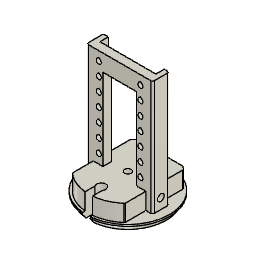
HANDLE_CONNECTOR v8 (Autodesk Fusion 360 design; units mm, degrees)
Autodesk Fusion 360 part; units mm, degrees
note: some values were not read from the file. Set by a fixed rule: which sketch regions a step uses.
sketch "Schizzo1" plane through (0, 0, 0) normal (0, 0, 1) x (1, 0, 0)
  circle A0 centre (0, 0) radius 25
  line L0 (0, 0) -> (0, 25) construction
  line L1 (0, 0) -> (0, -25) construction
  line L2 (-15.8, 19.3742) -> (-15.8, 17.5305) construction
  line L3 (-15.8, 17.5305) -> (-15.8, -17.5305)
  line L4 (-15.8, -17.5305) -> (-15.8, -19.3742) construction
  line L5 (15.8, 19.3742) -> (15.8, 17.5305) construction
  line L6 (15.8, 17.5305) -> (15.8, -17.5305)
  line L7 (15.8, -17.5305) -> (15.8, -19.3742) construction
  arc A1 (15.8, 17.5305) -> (-15.8, 17.5305) centre (0, 0) ccw
  arc A2 (-15.8, -17.5305) -> (15.8, -17.5305) centre (0, 0) ccw
  line L8 (-15.8, 0) -> (-19.8, 0) construction
  line L9 (15.8, 0) -> (19.8, 0) construction
  line L10 (-19.8, 0) -> (-19.8, 5)
  line L11 (-19.8, 5) -> (-15.8, 5)
  line L12 (-19.8, 0) -> (-19.8, -5)
  line L13 (-19.8, -5) -> (-15.8, -5)
  line L14 (19.8, 0) -> (19.8, 5)
  line L15 (19.8, 5) -> (15.8, 5)
  line L16 (19.8, 0) -> (19.8, -5)
  line L17 (19.8, -5) -> (15.8, -5)
  circle A3 centre (0, 0) radius 2
  circle A4 centre (0, -16) radius 2.75
  circle A5 centre (0, 10) radius 2
  line L18 (13.723, 19.2) -> (-13.723, 19.2)
  line L19 (2.25, -17.5811) -> (2.25, -24.8985)
  line L20 (-2.25, -17.5811) -> (-2.25, -24.8985)
  dimension "d1" = 50
  dimension "d3" = 31.6
  dimension "d4" = 1.4
  dimension "d5" = 10
  dimension "d6" = 4
  dimension "d21" = 4
  dimension "d22" = 5.5
  dimension "d23" = 16
  dimension "d39" = 4
  dimension "d40" = 10
  dimension "d45" = 5.8
  dimension "d48" = 4.5
  constraint coincident A0.centre L0.start
  constraint coincident A0 L0.end
  constraint vertical L0
  constraint coincident A0 L1.end
  constraint parallel L0 L1
  constraint coincident A0 L2.start
  constraint vertical L2
  constraint parallel L2 L3
  constraint coincident A0 L4.end
  constraint parallel L3 L4
  constraint coincident A0 L5.start
  constraint parallel L0 L5
  constraint parallel L5 L6
  constraint coincident A0 L7.end
  constraint parallel L6 L7
  constraint equal L5 L7
  constraint equal L2 L4
  constraint equal L2 L5
  constraint equal L3 L6
  constraint midpoint L3 L8.start
  constraint perpendicular L3 L8
  constraint midpoint L6 L9.start
  constraint perpendicular L6 L9
  constraint perpendicular L8 L10
  constraint coincident L3 L11.end
  constraint perpendicular L3 L11
  constraint perpendicular L8 L12
  constraint coincident L3 L13.end
  constraint perpendicular L3 L13
  constraint perpendicular L9 L14
  constraint coincident L6 L15.end
  constraint perpendicular L6 L15
  constraint perpendicular L9 L16
  constraint coincident L6 L17.end
  constraint perpendicular L6 L17
  constraint equal L10 L12
  constraint equal L14 L16
  constraint equal L12 L16
  constraint equal L8 L9
  constraint concentric A1 A3
  constraint coincident L1 A4.centre
  constraint coincident L0 A5.centre
  constraint coincident A1 L18.start
  constraint coincident A1 L18.end
  constraint perpendicular L6 L18
  constraint coincident A4 L19.start
  constraint coincident A0 L19.end
  constraint vertical L19
  constraint coincident A4 L20.start
  constraint coincident A0 L20.end
  constraint parallel L19 L20
  constraint equal L19 L20
  measures "d1" diameter of A0
  measures "d3" distance of L3 L6
  measures "d4" distance of A0 A1
  measures "d5" distance of L11 L13
  measures "d6" distance of L8.start L8.end
  measures "d21" diameter of A3
  measures "d22" diameter of A4
  measures "d23" distance of A0.centre A4.centre
  measures "d39" diameter of A5
  measures "d40" distance of A0.centre A5.centre
  measures "d45" distance of L0.end L18
  measures "d48" distance of L19 L20
extrude "Estrusione1" add sketch "Schizzo1" along normal blind 10 contours L3 L6 A1 A2 A4 L18 L19 L20 | L3 L10 L11 L12 L13 | L6 L14 L15 L16 L17
extrude "Estrusione2" add sketch "Schizzo1" against normal blind 4 contours A0 L3 L6 A1 A2 L10 L11 L12 L13 L14 L15 L16 L17 L19 L20 | L3 L6 A1 A2 A4 L18 L19 L20 | L3 L10 L11 L12 L13 | L6 L14 L15 L16 L17 | A1 L18
sketch "Schizzo2" plane through (-19.8, 0, 0) normal (-1, 0, 0) x (0, -1, 0)
  line L0 (-5, 0) -> (5, 0)
  line L1 (5, 0) -> (5, 10)
  line L2 (5, 10) -> (-5, 10)
  line L3 (-5, 10) -> (-5, 0)
  line L4 (0, 0) -> (0, 6.2) construction
  circle A0 centre (0, 6.2) radius 2
  dimension "d11" = 6.2
  dimension "d12" = 4
  constraint coincident L4.start origin
  constraint perpendicular L0 L4
  constraint coincident L4.end A0.centre
  measures "d11" distance of L4.start L4.end
  measures "d12" diameter of A0
extrude "Estrusione3" cut sketch "Schizzo2" against normal blind 15 contours A0
sketch "Schizzo3" plane through (19.8, 0, 0) normal (1, 0, 0) x (0, 1, 0)
  line L0 (-5, 0) -> (5, 0)
  line L1 (5, 0) -> (5, 10)
  line L2 (5, 10) -> (-5, 10)
  line L3 (-5, 10) -> (-5, 0)
  circle A0 centre (0, 6.2) radius 2
  circle A1 centre (0, 6.2) radius 2
extrude "Estrusione4" cut sketch "Schizzo3" against normal blind 15 contours A0 A1
chamfer "Smusso1" distance 1 angle 45 2 edges at (0, -13.25, -4) (-1.8647, -0.7232, -4)
chamfer "Smusso3" distance 2 distance2 3 1 edges at (0, 25, -4) measured on face at (-8.7268, -9.7213, -4)
fillet "Raccordo1" radius 2 1 edges at (-1.8647, -0.7232, -3)
sketch "Schizzo7" plane through (0, 0, 10) normal (0, 0, 1) x (-1, 0, 0)
  circle A0 centre (0, 0) radius 2
  circle A1 centre (0, -10) radius 2
  line L0 (-2.25, 17.5811) -> (-2.25, 23.4925)
  arc A2 (-2.25, 23.4925) -> (-15.8, 17.5305) centre (0, 0) ccw
  line L1 (-15.8, 17.5305) -> (-15.8, 5)
  line L2 (-15.8, 5) -> (-19.8, 5)
  line L3 (-19.8, 5) -> (-19.8, -5)
  line L4 (-19.8, -5) -> (-15.8, -5)
  line L5 (-15.8, -5) -> (-15.8, -17.5305)
  arc A3 (-15.8, -17.5305) -> (-13.723, -19.2) centre (0, 0) ccw
  line L6 (-13.723, -19.2) -> (13.723, -19.2)
  arc A4 (13.723, -19.2) -> (15.8, -17.5305) centre (0, 0) ccw
  line L7 (15.8, -17.5305) -> (15.8, -5)
  line L8 (15.8, -5) -> (19.8, -5)
  line L9 (19.8, -5) -> (19.8, 5)
  line L10 (19.8, 5) -> (15.8, 5)
  line L11 (15.8, 5) -> (15.8, 17.5305)
  arc A5 (15.8, 17.5305) -> (2.25, 23.4925) centre (0, 0) ccw
  line L12 (2.25, 23.4925) -> (2.25, 17.5811)
  arc A6 (-2.25, 17.5811) -> (2.25, 17.5811) centre (0, 16) ccw
  line L13 (15.8, -5) -> (16.8, -5)
  line L14 (16.8, -5) -> (16.8, 0)
  line L15 (16.8, 0) -> (10, 0)
  line L16 (10, 0) -> (10, 5)
  line L17 (10, 5) -> (15.8, 5)
  line L18 (-15.8, -5) -> (-16.8, -5)
  line L19 (-16.8, -5) -> (-16.8, 0)
  line L20 (-16.8, 0) -> (-10, 0)
  line L21 (-10, 0) -> (-10, 5)
  line L22 (-10, 5) -> (-15.8, 5)
  dimension "d49" = 3
  dimension "d50" = 20
  dimension "d51" = 5
  constraint coincident L7.end L8.start
  constraint perpendicular L7 L13
  constraint perpendicular L8 L14
  constraint perpendicular L14 L15
  constraint perpendicular L15 L16
  constraint coincident L10.end L11.start
  constraint coincident L4.end L5.start
  constraint perpendicular L5 L18
  constraint perpendicular L4 L19
  constraint perpendicular L19 L20
  constraint perpendicular L4 L21
  constraint coincident L1.end L2.start
  constraint perpendicular L21 L22
  constraint perpendicular L16 L17
  constraint equal L17 L22
  constraint equal L16 L21
  constraint equal L15 L20
  measures "d49" distance of L9 L14
  measures "d50" distance of L16 L21
  measures "d51" distance of L15.end L16.end
extrude "Estrusione6" add sketch "Schizzo7" along normal blind 59 contours L2 L3 L4 L19 L20 L21 L22 | L8 L9 L10 L14 L15 L16 L17
sketch "Schizzo8" plane through (0, 0, 69) normal (0, 0, 1) x (-1, 0, 0)
  line L0 (16.8, -5) -> (19.8, -5)
  line L1 (19.8, -5) -> (19.8, 5)
  line L2 (19.8, 5) -> (10, 5)
  line L3 (10, 5) -> (10, 0)
  line L4 (10, 0) -> (16.8, 0)
  line L5 (16.8, 0) -> (16.8, -5)
  line L6 (-10, 5) -> (-19.8, 5)
  line L7 (-19.8, 5) -> (-19.8, -5)
  line L8 (-19.8, -5) -> (-16.8, -5)
  line L9 (-16.8, -5) -> (-16.8, 0)
  line L10 (-16.8, 0) -> (-10, 0)
  line L11 (-10, 0) -> (-10, 5)
  line L12 (-10, 5) -> (10, 5)
  line L13 (-10, 0) -> (10, 0)
  constraint coincident L6.start L11.end
  constraint coincident L2.end L3.start
  constraint coincident L10.end L11.start
  constraint coincident L3.end L4.start
extrude "Estrusione7" add sketch "Schizzo8" against normal blind 10 contours L3 L11 L12 L13
sketch "Schizzo9" plane through (0, 0, 0) normal (0, 1, 0) x (-1, 0, 0)
  line L0 (10, 10) -> (16.8, 10)
  line L1 (16.8, 10) -> (16.8, 69)
  line L2 (16.8, 69) -> (-16.8, 69)
  line L3 (-16.8, 69) -> (-16.8, 10)
  line L4 (-16.8, 10) -> (-10, 10)
  line L5 (-10, 10) -> (-10, 59)
  line L6 (-10, 59) -> (10, 59)
  line L7 (10, 59) -> (10, 10)
  line L8 (-12.5, 69) -> (-12.5, 10) construction
  line L9 (0, 69) -> (0, 59) construction
  line L10 (-13.4642, 40.6491) -> (-12.5, 41.4581)
  line L11 (-12.5, 41.4581) -> (-11.5358, 40.6491)
  arc A0 (-13.4642, 40.6491) -> (-11.5358, 40.6491) centre (-12.5, 39.5) ccw
  arc A1 (-13.4642, 16.6491) -> (-11.5358, 16.6491) centre (-12.5, 15.5) ccw
  line L12 (-12.5, 17.4581) -> (-11.5358, 16.6491)
  line L13 (-13.4642, 16.6491) -> (-12.5, 17.4581)
  arc A2 (11.5358, 16.6491) -> (13.4642, 16.6491) centre (12.5, 15.5) ccw
  line L14 (12.5, 17.4581) -> (13.4642, 16.6491)
  line L15 (11.5358, 16.6491) -> (12.5, 17.4581)
  arc A3 (-13.4642, 24.6491) -> (-11.5358, 24.6491) centre (-12.5, 23.5) ccw
  line L16 (-12.5, 25.4581) -> (-11.5358, 24.6491)
  line L17 (-13.4642, 24.6491) -> (-12.5, 25.4581)
  arc A4 (11.5358, 24.6491) -> (13.4642, 24.6491) centre (12.5, 23.5) ccw
  line L18 (12.5, 25.4581) -> (13.4642, 24.6491)
  line L19 (11.5358, 24.6491) -> (12.5, 25.4581)
  arc A5 (-13.4642, 32.6491) -> (-11.5358, 32.6491) centre (-12.5, 31.5) ccw
  line L20 (-12.5, 33.4581) -> (-11.5358, 32.6491)
  line L21 (-13.4642, 32.6491) -> (-12.5, 33.4581)
  arc A6 (11.5358, 32.6491) -> (13.4642, 32.6491) centre (12.5, 31.5) ccw
  line L22 (12.5, 33.4581) -> (13.4642, 32.6491)
  line L23 (11.5358, 32.6491) -> (12.5, 33.4581)
  arc A7 (11.5358, 40.6491) -> (13.4642, 40.6491) centre (12.5, 39.5) ccw
  line L24 (12.5, 41.4581) -> (13.4642, 40.6491)
  line L25 (11.5358, 40.6491) -> (12.5, 41.4581)
  arc A8 (-13.4642, 48.6491) -> (-11.5358, 48.6491) centre (-12.5, 47.5) ccw
  line L26 (-12.5, 49.4581) -> (-11.5358, 48.6491)
  line L27 (-13.4642, 48.6491) -> (-12.5, 49.4581)
  arc A9 (11.5358, 48.6491) -> (13.4642, 48.6491) centre (12.5, 47.5) ccw
  line L28 (12.5, 49.4581) -> (13.4642, 48.6491)
  line L29 (11.5358, 48.6491) -> (12.5, 49.4581)
  arc A10 (-13.4642, 56.6491) -> (-11.5358, 56.6491) centre (-12.5, 55.5) ccw
  line L30 (-12.5, 57.4581) -> (-11.5358, 56.6491)
  line L31 (-13.4642, 56.6491) -> (-12.5, 57.4581)
  arc A11 (11.5358, 56.6491) -> (13.4642, 56.6491) centre (12.5, 55.5) ccw
  line L32 (12.5, 57.4581) -> (13.4642, 56.6491)
  line L33 (11.5358, 56.6491) -> (12.5, 57.4581)
  arc A12 (-13.4642, 64.6491) -> (-11.5358, 64.6491) centre (-12.5, 63.5) ccw
  line L34 (-12.5, 65.4581) -> (-11.5358, 64.6491)
  line L35 (-13.4642, 64.6491) -> (-12.5, 65.4581)
  arc A13 (11.5358, 64.6491) -> (13.4642, 64.6491) centre (12.5, 63.5) ccw
  line L36 (12.5, 65.4581) -> (13.4642, 64.6491)
  line L37 (11.5358, 64.6491) -> (12.5, 65.4581)
  dimension "d57" = 12.5
  dimension "d58" = 50
  dimension "d59" = 1.5
  dimension "d62" = 25
  dimension "d63" = 8
  constraint coincident L2 L8.start
  constraint coincident L4 L8.end
  constraint perpendicular L2 L8
  constraint midpoint L2 L9.start
  constraint midpoint L6 L9.end
  constraint coincident L8 L10.end
  constraint midpoint L8 A0.centre
  constraint tangent L10 A0
  constraint tangent L11 A0
  measures "d57" distance of L8 L9
  measures "d58" angle of L8 L10
  measures "d59" radius of A0
extrude "Estrusione8" cut sketch "Schizzo9" against normal blind 5 contours L10 L11 A0 | A1 L12 L13 | A2 L14 L15 | A3 L16 L17 | A4 L18 L19 | A5 L20 L21 | A6 L22 L23 | A7 L24 L25 | A8 L26 L27 | A9 L28 L29 | A10 L30 L31 | A11 L32 L33 | A12 L34 L35 | A13 L36 L37
fillet "Raccordo5" radius 1 4 edges at (19.8, -5, 34.5) (19.8, 5, 34.5) (-19.8, -5, 34.5) (-19.8, 5, 34.5)
fillet "Raccordo6" radius 1 6 edges at (15.8, -17.5305, 5) (13.723, 19.2, 5) (15.8, 17.5305, 5) (-15.8, 17.5305, 5) (-13.723, 19.2, 5) (-15.8, -17.5305, 5)
component "Component" placed x (1, 0, 0) y (0, 1, 0) z (0, 0, 1) at (0, 0, 0)
